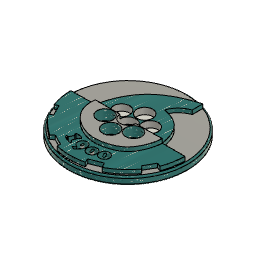
Pin (Autodesk Fusion 360 design; units mm, degrees)
Autodesk Fusion 360 part; units mm, degrees
cylinder "CylinderPrimitive1" add diameter 15 height 1 placed x (1, 0, 0) y (0, 1, 0) z (0, 0, 1) at (0, 0, 0)
fillet "Fillet1" radius 0.2 1 edges at (-6.9925, -2.7121, 1)
fillet "Fillet2" radius 0.2 1 edges at (-6.9925, 2.7121, 0)
shell "Shell1" thickness 0.3 removed faces 0 bodies 1
cylinder "CylinderPrimitive2" cut diameter 2 height 1 placed x (1, 0, 0) y (0, 1, 0) z (0, 0, 1) at (0, 0, 0.3)
cylinder "CylinderPrimitive3" cut diameter 2 height -0.3 placed x (1, 0, 0) y (0, 1, 0) z (0, 0, 1) at (-0.0026, -2.1739, 1)
cylinder "CylinderPrimitive4" cut diameter 2 height -0.3 placed x (1, 0, 0) y (0, 1, 0) z (0, 0, 1) at (-1.832, 1.0276, 1)
cylinder "CylinderPrimitive5" cut diameter 2 height -0.3 placed x (1, 0, 0) y (0, 1, 0) z (0, 0, 1) at (-1.832, -1.0481, 1)
cylinder "CylinderPrimitive6" cut diameter 2 height -0.3 placed x (1, 0, 0) y (0, 1, 0) z (0, 0, 1) at (0, 2.1, 1)
cylinder "CylinderPrimitive7" cut diameter 2 height -0.3 placed x (1, 0, 0) y (0, 1, 0) z (0, 0, 1) at (1.8, 1, 1)
cylinder "CylinderPrimitive8" cut diameter 2 height -0.3 placed x (1, 0, 0) y (0, 1, 0) z (0, 0, 1) at (1.8, -1.1, 1)
cylinder "CylinderPrimitive9" cut diameter 1.25 height -0.3 placed x (1, 0, 0) y (0, 1, 0) z (0, 0, 1) at (1.9983, -4.9501, 1)
sketch "Sketch22" plane through (0, 0, 0.3) normal (0, 0, 1) x (-1, 0, 0)
  circle A0 centre (0, 0) radius 7.2
  ellipse E0 centre (-2.0085, 4.9449) end of major axis (-2.1682, 5.2369) minor radius 0.1458
  line L0 (-1.8488, 4.6529) -> (-2.1682, 5.2369)
  line L1 (-1.8806, 5.0149) -> (-2.1365, 4.8749)
  constraint coincident E0 L0.start
  constraint coincident E0 L0.end
  constraint coincident E0 L1.start
  constraint coincident E0 L1.end
extrude "Extrude1" add sketch "Sketch22" along normal blind 0.7 contours E0 L0 L1 | E0 L0 L1 | E0 L0 L1 | E0 L0 L1
cylinder "CylinderPrimitive10" cut diameter 1.25 height -0.3 placed x (1, 0, 0) y (0, 1, 0) z (0, 0, 1) at (0.7297, -5.2531, 1)
sketch "Sketch24" plane through (0, 0, 0.3) normal (0, 0, 1) x (-1, 0, 0)
  ellipse E0 centre (-2.0085, 4.9449) end of major axis (-2.1682, 5.2369) minor radius 0.1458
  circle A0 centre (0, 0) radius 7.2
  ellipse E1 centre (-0.7296, 5.2552) end of major axis (-0.8009, 5.5528) minor radius 0.1336
  line L0 (-0.6584, 4.9577) -> (-0.8009, 5.5528)
  line L1 (-0.5997, 5.2863) -> (-0.8596, 5.2241)
  constraint coincident E1 L0.start
  constraint coincident E1 L0.end
  constraint coincident E1 L1.start
  constraint coincident E1 L1.end
extrude "Extrude2" add sketch "Sketch24" along normal blind 0.7 contours E1 L0 L1 | E1 L0 L1 | E1 L0 L1 | E1 L0 L1
cylinder "CylinderPrimitive11" cut diameter 1.175 height -0.3 placed x (1, 0, 0) y (0, 1, 0) z (0, 0, 1) at (-0.5634, -5.1632, 1)
sketch "Sketch26" plane through (0, 0, 0.3) normal (0, 0, 1) x (-1, 0, 0)
  ellipse E0 centre (-0.7296, 5.2552) end of major axis (-0.8009, 5.5528) minor radius 0.1336
  ellipse E1 centre (-2.0085, 4.9449) end of major axis (-2.1682, 5.2369) minor radius 0.1458
  circle A0 centre (0, 0) radius 7.2
  ellipse E2 centre (0.5487, 5.1901) end of major axis (0.5487, 5.4) minor radius 0.1259
  line L0 (0.5487, 4.9802) -> (0.5487, 5.4)
  line L1 (0.6746, 5.1901) -> (0.4229, 5.1901)
  constraint vertical L0
  constraint coincident E2 L0.start
  constraint coincident E2 L0.end
  constraint coincident E2 L1.start
  constraint coincident E2 L1.end
extrude "Extrude3" add sketch "Sketch26" along normal blind 0.7 contours E2 L0 L1 | E2 L0 L1 | E2 L0 L1 | E2 L0 L1
sketch "Sketch27" plane through (0, 0, 1) normal (0, 0, 1) x (-1, 0, 0)
  circle A0 centre (0.5634, 5.1632) radius 0.5875
  circle A1 centre (-0.7297, 5.2531) radius 0.625
  circle A2 centre (-1.9983, 4.9501) radius 0.625
  circle A3 centre (-1.8, 1.1) radius 1
  circle A4 centre (-1.8, -1) radius 1
  circle A5 centre (0, -2.1) radius 1
  circle A6 centre (1.832, 1.0481) radius 1
  circle A7 centre (1.832, -1.0276) radius 1
  circle A8 centre (0.0026, 2.1739) radius 1
  circle A9 centre (0, 0) radius 1
  circle A10 centre (0, 0) radius 7.3
  spline S0 degree 5 poles (0.014, 5.3712) (0.023, 5.3959) (0.0414, 5.4447) (0.0703, 5.5157) (0.1114, 5.6061) (0.1671, 5.7113) (0.2276, 5.8082) (0.2934, 5.896) (0.3646, 5.9743) (0.4412, 6.0434) (0.5227, 6.1039) (0.5915, 6.146) (0.645, 6.1743) (0.6815, 6.1917) (0.7, 6.2) knots 0 0 0 0 0 0 0.1 0.2 0.3 0.4 0.5 0.6 0.7 0.8 0.9 1 1 1 1 1 1
  spline S1 degree 5 poles (0.7, 5.7346) (0.7041, 5.7419) (0.7123, 5.7564) (0.7253, 5.7775) (0.7435, 5.8047) (0.7682, 5.8367) (0.7949, 5.8666) (0.8238, 5.8943) (0.8549, 5.9197) (0.8882, 5.9428) (0.9235, 5.9639) (0.9533, 5.9792) (0.9763, 5.9899) (0.9921, 5.9967) (1, 6) knots 0 0 0 0 0 0 0.1 0.2 0.3 0.4 0.5 0.6 0.7 0.8 0.9 1 1 1 1 1 1
  line L0 (0.7, 6.2) -> (1, 6)
  point P0 (0.3, 5.9)
  point P1 (0.8243, 5.8937)
  constraint coincident A0 S0.start
  constraint coincident A0 S1.start
extrude "Extrude4" cut sketch "Sketch27" against normal blind 0.3 contours A0 S0 S1 L0
sketch "Sketch28" plane through (0, 0, 1) normal (0, 0, 1) x (-1, 0, 0)
  spline S0 degree 5 poles (1, 6) (0.9921, 5.9967) (0.9763, 5.9899) (0.9533, 5.9792) (0.9235, 5.9639) (0.8882, 5.9428) (0.8549, 5.9197) (0.8238, 5.8943) (0.7949, 5.8666) (0.7682, 5.8367) (0.7435, 5.8047) (0.7253, 5.7775) (0.7123, 5.7564) (0.7041, 5.7419) (0.7, 5.7346) knots -1 -1 -1 -1 -1 -1 -0.9 -0.8 -0.7 -0.6 -0.5 -0.4 -0.3 -0.2 -0.1 0 0 0 0 0 0
  arc A0 (0.014, 5.3712) -> (0.7, 5.7346) centre (0.5634, 5.1632) ccw
  spline S1 degree 5 poles (0.014, 5.3712) (0.023, 5.3959) (0.0414, 5.4447) (0.0703, 5.5157) (0.1114, 5.6061) (0.1671, 5.7113) (0.2276, 5.8082) (0.2934, 5.896) (0.3646, 5.9743) (0.4412, 6.0434) (0.5227, 6.1039) (0.5915, 6.146) (0.645, 6.1743) (0.6815, 6.1917) (0.7, 6.2) knots 0 0 0 0 0 0 0.1 0.2 0.3 0.4 0.5 0.6 0.7 0.8 0.9 1 1 1 1 1 1
  line L0 (0.7, 6.2) -> (1, 6)
  circle A1 centre (-0.7297, 5.2531) radius 0.625
  circle A2 centre (-1.9983, 4.9501) radius 0.625
  circle A3 centre (-1.8, 1.1) radius 1
  circle A4 centre (-1.8, -1) radius 1
  circle A5 centre (0, -2.1) radius 1
  circle A6 centre (1.832, 1.0481) radius 1
  circle A7 centre (1.832, -1.0276) radius 1
  circle A8 centre (0.0026, 2.1739) radius 1
  circle A9 centre (0, 0) radius 1
  circle A10 centre (0, 0) radius 7.3
  spline S2 degree 5 poles (2.1731, 4.3495) (2.1626, 4.3461) (2.1405, 4.3398) (2.1042, 4.3322) (2.0494, 4.3261) (1.9705, 4.325) (1.8818, 4.3305) (1.785, 4.3423) (1.6831, 4.3601) (1.5808, 4.3831) (1.4843, 4.4103) (1.3999, 4.4405) (1.3336, 4.4724) (1.2892, 4.5048) (1.2683, 4.5365) (1.2686, 4.5667) (1.2857, 4.5947) (1.3144, 4.6201) (1.3495, 4.6426) (1.3872, 4.6619) (1.4255, 4.6781) (1.4557, 4.6884) (1.478, 4.6948) (1.4927, 4.6984) (1.5, 4.7) knots 0 0 0 0 0 0 0.05 0.1 0.15 0.2 0.25 0.3 0.35 0.4 0.45 0.5 0.55 0.6 0.65 0.7 0.75 0.8 0.85 0.9 0.95 1 1 1 1 1 1
  line L1 (1.5, 4.7) -> (1.7, 5.3)
  spline S3 degree 5 poles (1.7, 5.3) (1.7086, 5.3088) (1.7237, 5.3259) (1.7404, 5.3504) (1.7508, 5.3807) (1.7442, 5.4149) (1.7194, 5.4456) (1.6794, 5.4737) (1.6295, 5.5008) (1.5772, 5.5288) (1.5309, 5.5592) (1.4986, 5.5926) (1.4873, 5.628) (1.5016, 5.6619) (1.5434, 5.6892) (1.6127, 5.7046) (1.7069, 5.7036) (1.8216, 5.6836) (1.95, 5.6454) (2.084, 5.592) (2.2151, 5.5276) (2.3346, 5.4577) (2.4346, 5.3876) (2.5084, 5.3218) (2.5517, 5.2637) (2.5622, 5.2152) (2.5436, 5.1847) (2.5144, 5.1665) (2.4882, 5.1565) (2.4734, 5.1521) knots 0 0 0 0 0 0 0.04 0.08 0.12 0.16 0.2 0.24 0.28 0.32 0.36 0.4 0.44 0.48 0.52 0.56 0.6 0.64 0.68 0.72 0.76 0.8 0.84 0.88 0.92 0.96 1 1 1 1 1 1
  line L2 (2.4734, 5.1521) -> (2.3, 5.2)
  line L3 (2.3, 5.2) -> (2.0366, 4.6553)
  spline S4 degree 5 poles (2.0366, 4.6553) (2.0437, 4.6504) (2.0575, 4.6406) (2.0771, 4.6256) (2.1009, 4.6049) (2.1265, 4.5778) (2.1476, 4.5493) (2.1638, 4.5195) (2.1749, 4.4882) (2.1811, 4.4555) (2.1828, 4.4214) (2.1809, 4.3932) (2.1777, 4.3716) (2.1748, 4.3569) (2.1731, 4.3495) knots 0 0 0 0 0 0 0.1 0.2 0.3 0.4 0.5 0.6 0.7 0.8 0.9 1 1 1 1 1 1
  point P0 (1.7473, 4.3495)
  point P1 (1.3, 4.5)
  point P2 (1.3269, 4.6272)
  point P3 (1.7, 5.4578)
  point P4 (1.5, 5.6)
  point P5 (1.7, 5.7)
  point P6 (2.457, 5.365)
  point P7 (2.1627, 4.5186)
extrude "Extrude5" cut sketch "Sketch28" against normal blind 0.3 contours S2 L1 S3 L2 L3 S4
sketch "Sketch29" plane through (0, 0, 1) normal (0, 0, 1) x (-1, 0, 0)
  line L0 (2.4734, 5.1521) -> (2.3, 5.2)
  line L1 (2.3, 5.2) -> (2.0366, 4.6553)
  spline S0 degree 5 poles (2.0366, 4.6553) (2.0437, 4.6504) (2.0575, 4.6406) (2.0771, 4.6256) (2.1009, 4.6049) (2.1265, 4.5778) (2.1476, 4.5493) (2.1638, 4.5195) (2.1749, 4.4882) (2.1811, 4.4555) (2.1828, 4.4214) (2.1809, 4.3932) (2.1777, 4.3716) (2.1748, 4.3569) (2.1731, 4.3495) knots 0 0 0 0 0 0 0.1 0.2 0.3 0.4 0.5 0.6 0.7 0.8 0.9 1 1 1 1 1 1
  spline S1 degree 5 poles (2.1731, 4.3495) (2.1626, 4.3461) (2.1405, 4.3398) (2.1042, 4.3322) (2.0494, 4.3261) (1.9705, 4.325) (1.8818, 4.3305) (1.785, 4.3423) (1.6831, 4.3601) (1.5808, 4.3831) (1.4843, 4.4103) (1.3999, 4.4405) (1.3336, 4.4724) (1.2892, 4.5048) (1.2683, 4.5365) (1.2686, 4.5667) (1.2857, 4.5947) (1.3144, 4.6201) (1.3495, 4.6426) (1.3872, 4.6619) (1.4255, 4.6781) (1.4557, 4.6884) (1.478, 4.6948) (1.4927, 4.6984) (1.5, 4.7) knots 0 0 0 0 0 0 0.05 0.1 0.15 0.2 0.25 0.3 0.35 0.4 0.45 0.5 0.55 0.6 0.65 0.7 0.75 0.8 0.85 0.9 0.95 1 1 1 1 1 1
  line L2 (1.5, 4.7) -> (1.7, 5.3)
  spline S2 degree 5 poles (1.7, 5.3) (1.7086, 5.3088) (1.7237, 5.3259) (1.7404, 5.3504) (1.7508, 5.3807) (1.7442, 5.4149) (1.7194, 5.4456) (1.6794, 5.4737) (1.6295, 5.5008) (1.5772, 5.5288) (1.5309, 5.5592) (1.4986, 5.5926) (1.4873, 5.628) (1.5016, 5.6619) (1.5434, 5.6892) (1.6127, 5.7046) (1.7069, 5.7036) (1.8216, 5.6836) (1.95, 5.6454) (2.084, 5.592) (2.2151, 5.5276) (2.3346, 5.4577) (2.4346, 5.3876) (2.5084, 5.3218) (2.5517, 5.2637) (2.5622, 5.2152) (2.5436, 5.1847) (2.5144, 5.1665) (2.4882, 5.1565) (2.4734, 5.1521) knots 0 0 0 0 0 0 0.04 0.08 0.12 0.16 0.2 0.24 0.28 0.32 0.36 0.4 0.44 0.48 0.52 0.56 0.6 0.64 0.68 0.72 0.76 0.8 0.84 0.88 0.92 0.96 1 1 1 1 1 1
  spline S3 degree 5 poles (1, 6) (0.9921, 5.9967) (0.9763, 5.9899) (0.9533, 5.9792) (0.9235, 5.9639) (0.8882, 5.9428) (0.8549, 5.9197) (0.8238, 5.8943) (0.7949, 5.8666) (0.7682, 5.8367) (0.7435, 5.8047) (0.7253, 5.7775) (0.7123, 5.7564) (0.7041, 5.7419) (0.7, 5.7346) knots -1 -1 -1 -1 -1 -1 -0.9 -0.8 -0.7 -0.6 -0.5 -0.4 -0.3 -0.2 -0.1 0 0 0 0 0 0
  arc A0 (0.014, 5.3712) -> (0.7, 5.7346) centre (0.5634, 5.1632) ccw
  spline S4 degree 5 poles (0.014, 5.3712) (0.023, 5.3959) (0.0414, 5.4447) (0.0703, 5.5157) (0.1114, 5.6061) (0.1671, 5.7113) (0.2276, 5.8082) (0.2934, 5.896) (0.3646, 5.9743) (0.4412, 6.0434) (0.5227, 6.1039) (0.5915, 6.146) (0.645, 6.1743) (0.6815, 6.1917) (0.7, 6.2) knots 0 0 0 0 0 0 0.1 0.2 0.3 0.4 0.5 0.6 0.7 0.8 0.9 1 1 1 1 1 1
  line L3 (0.7, 6.2) -> (1, 6)
  circle A1 centre (-0.7297, 5.2531) radius 0.625
  circle A2 centre (-1.9983, 4.9501) radius 0.625
  circle A3 centre (-1.8, 1.1) radius 1
  circle A4 centre (-1.8, -1) radius 1
  circle A5 centre (0, -2.1) radius 1
  circle A6 centre (1.832, 1.0481) radius 1
  circle A7 centre (1.832, -1.0276) radius 1
  circle A8 centre (0.0026, 2.1739) radius 1
  circle A9 centre (0, 0) radius 1
  circle A10 centre (0, 0) radius 7.3
  spline S5 degree 5 poles (4.13, -0.0103) (4.0869, -0.2194) (3.9925, -0.6311) (3.8269, -1.2295) (3.5572, -1.9883) (3.1331, -2.8673) (2.6146, -3.6709) (1.9943, -4.3931) (1.2689, -5.0314) (0.4435, -5.5897) (-0.4741, -6.0744) (-1.2757, -6.4081) (-1.9125, -6.63) (-2.3525, -6.7656) (-2.5765, -6.8302) knots 0 0 0 0 0 0 0.1 0.2 0.3 0.4 0.5 0.6 0.7 0.8 0.9 1 1 1 1 1 1
  line L4 (-2.5765, -6.8302) -> (-2.5765, -5.5)
  spline S6 degree 5 poles (-2.5765, -5.5) (-2.5232, -5.4786) (-2.4184, -5.4346) (-2.266, -5.3651) (-2.0727, -5.2656) (-1.8485, -5.1288) (-1.6435, -4.9784) (-1.4591, -4.8134) (-1.2965, -4.633) (-1.1549, -4.4377) (-1.0327, -4.2287) (-0.9493, -4.0513) (-0.8943, -3.913) (-0.8609, -3.8184) (-0.845, -3.7705) knots 0 0 0 0 0 0 0.1 0.2 0.3 0.4 0.5 0.6 0.7 0.8 0.9 1 1 1 1 1 1
  spline S7 degree 5 poles (-0.845, -3.7705) (-0.9645, -3.747) (-1.1989, -3.6953) (-1.5374, -3.6041) (-1.9618, -3.4547) (-2.4443, -3.2186) (-2.8747, -2.9286) (-3.2489, -2.5806) (-3.5648, -2.1724) (-3.8249, -1.7066) (-4.0335, -1.1877) (-4.1627, -0.7337) (-4.2397, -0.3726) (-4.2824, -0.1229) (-4.3015, 0.0041) knots 0 0 0 0 0 0 0.1 0.2 0.3 0.4 0.5 0.6 0.7 0.8 0.9 1 1 1 1 1 1
  line L5 (-4.3015, 0.0041) -> (-7.1651, 0.0041)
  spline S8 degree 5 poles (-7.1651, 0.0041) (-7.1621, 0.0669) (-7.1557, 0.1917) (-7.1441, 0.3763) (-7.125, 0.6172) (-7.0942, 0.9092) (-7.0561, 1.191) (-7.01, 1.4618) (-6.9555, 1.7211) (-6.8927, 1.969) (-6.8222, 2.2065) (-6.7602, 2.3887) (-6.7107, 2.5213) (-6.6764, 2.6079) (-6.6589, 2.6507) knots 0 0 0 0 0 0 0.1 0.2 0.3 0.4 0.5 0.6 0.7 0.8 0.9 1 1 1 1 1 1
  line L6 (-6.6589, 2.6507) -> (-6.1816, 2.4772)
  line L7 (-6.1816, 2.4772) -> (-5.473, 3.7354)
  line L8 (-5.473, 3.7354) -> (-5.8273, 4.1259)
  spline S9 degree 5 poles (-5.8273, 4.1259) (-5.7769, 4.187) (-5.6759, 4.3077) (-5.5236, 4.4848) (-5.3192, 4.7127) (-5.0612, 4.9829) (-4.8005, 5.2371) (-4.5368, 5.4739) (-4.2699, 5.6923) (-4, 5.8929) (-3.7272, 6.0769) (-3.5069, 6.2118) (-3.3406, 6.3066) (-3.2293, 6.367) (-3.1735, 6.3965) knots 0 0 0 0 0 0 0.1 0.2 0.3 0.4 0.5 0.6 0.7 0.8 0.9 1 1 1 1 1 1
  line L9 (-3.1735, 6.3965) -> (-2.8264, 5.8035)
  line L10 (-2.8264, 5.8035) -> (-1.3367, 6.3965)
  line L11 (-1.3367, 6.3965) -> (-1.5394, 6.9057)
  spline S10 degree 5 poles (-1.5394, 6.9057) (-1.4688, 6.9219) (-1.3277, 6.9529) (-1.1159, 6.9952) (-0.8336, 7.043) (-0.4807, 7.0873) (-0.1277, 7.1149) (0.2252, 7.1243) (0.5781, 7.1149) (0.931, 7.0873) (1.2838, 7.043) (1.5662, 6.9952) (1.7779, 6.9529) (1.919, 6.9219) (1.9896, 6.9057) knots 0 0 0 0 0 0 0.1 0.2 0.3 0.4 0.5 0.6 0.7 0.8 0.9 1 1 1 1 1 1
  line L12 (1.9896, 6.9057) -> (1.9896, 6.5)
  line L13 (1.9896, 6.5) -> (3.2912, 5.8469)
  line L14 (3.2912, 5.8469) -> (3.6817, 6.1735)
  spline S11 degree 5 poles (3.6817, 6.1735) (3.7466, 6.1256) (3.8748, 6.0303) (4.0624, 5.8884) (4.3029, 5.7015) (4.5865, 5.472) (4.8512, 5.2469) (5.0953, 5.0266) (5.3175, 4.8115) (5.5182, 4.6016) (5.6985, 4.3964) (5.8279, 4.2358) (5.917, 4.1172) (5.9729, 4.0389) (6, 4) knots 0 0 0 0 0 0 0.1 0.2 0.3 0.4 0.5 0.6 0.7 0.8 0.9 1 1 1 1 1 1
  line L15 (6, 4) -> (5.5907, 3.7354)
  line L16 (5.5907, 3.7354) -> (6.2849, 2.3904)
  line L17 (6.2849, 2.3904) -> (6.6861, 2.5975)
  spline S12 degree 5 poles (6.6861, 2.5975) (6.705, 2.5422) (6.7421, 2.432) (6.7951, 2.2677) (6.8608, 2.0505) (6.9339, 1.7825) (6.9971, 1.5182) (7.0496, 1.2581) (7.0909, 1.0023) (7.1213, 0.7506) (7.1415, 0.5029) (7.1503, 0.3075) (7.153, 0.1625) (7.1531, 0.0664) (7.1527, 0.0186) knots 0 0 0 0 0 0 0.1 0.2 0.3 0.4 0.5 0.6 0.7 0.8 0.9 1 1 1 1 1 1
  line L18 (7.1527, 0.0186) -> (4.13, -0.0103)
  point P0 (2.033, -4.3057)
  point P1 (-1.4524, -4.7974)
  point P2 (-3.2168, -2.5846)
  point P3 (-7, 1.5)
  point P4 (-4.5, 5.5)
  point P5 (0.2252, 7.1196)
  point P6 (5.1569, 4.9647)
  point P7 (7.0514, 1.2334)
  constraint coincident A10 S5.end
  constraint vertical L4
  constraint horizontal L5
  constraint perpendicular L10 L11
  constraint vertical L12
  constraint perpendicular L16 L17
extrude "Extrude6" add sketch "Sketch29" along normal blind 0.5 contours S5 L4 S6 S7 L5 S8 L6 L7 L8 S9 L9 L10 L11 S10 L12 L13 L14 S11 L15 L16 L17 S12 L18
extrude "Extrude7" add 1 faces at (-0.5898, -5.2144, 1) along direction (0, 0, 1) blind 0.5
extrude "Extrude8" add 1 faces at (0.697, -5.3058, 1) along direction (0, 0, 1) blind 0.5
extrude "Extrude9" add 1 faces at (2.0285, -4.8824, 1) along direction (0, 0, 1) blind 0.5
sketch "Sketch31" plane through (0, 0, 1.5) normal (0, 0, 1) x (-1, 0, 0)
  arc A0 (0.014, 5.3712) -> (0.7, 5.7346) centre (0.5634, 5.1632) ccw
  spline S0 degree 5 poles (0.014, 5.3712) (0.023, 5.3959) (0.0414, 5.4447) (0.0703, 5.5157) (0.1114, 5.6061) (0.1671, 5.7113) (0.2276, 5.8082) (0.2934, 5.896) (0.3646, 5.9743) (0.4412, 6.0434) (0.5227, 6.1039) (0.5915, 6.146) (0.645, 6.1743) (0.6815, 6.1917) (0.7, 6.2) knots 0 0 0 0 0 0 0.1 0.2 0.3 0.4 0.5 0.6 0.7 0.8 0.9 1 1 1 1 1 1
  line L0 (0.7, 6.2) -> (1, 6)
  spline S1 degree 5 poles (1, 6) (0.9921, 5.9967) (0.9763, 5.9899) (0.9533, 5.9792) (0.9235, 5.9639) (0.8882, 5.9428) (0.8549, 5.9197) (0.8238, 5.8943) (0.7949, 5.8666) (0.7682, 5.8367) (0.7435, 5.8047) (0.7253, 5.7775) (0.7123, 5.7564) (0.7041, 5.7419) (0.7, 5.7346) knots -1 -1 -1 -1 -1 -1 -0.9 -0.8 -0.7 -0.6 -0.5 -0.4 -0.3 -0.2 -0.1 0 0 0 0 0 0
  circle A1 centre (0, 0) radius 1
  line L1 (1.5, 4.7) -> (1.7, 5.3)
  spline S2 degree 5 poles (1.7, 5.3) (1.7086, 5.3088) (1.7237, 5.3259) (1.7404, 5.3504) (1.7508, 5.3807) (1.7442, 5.4149) (1.7194, 5.4456) (1.6794, 5.4737) (1.6295, 5.5008) (1.5772, 5.5288) (1.5309, 5.5592) (1.4986, 5.5926) (1.4873, 5.628) (1.5016, 5.6619) (1.5434, 5.6892) (1.6127, 5.7046) (1.7069, 5.7036) (1.8216, 5.6836) (1.95, 5.6454) (2.084, 5.592) (2.2151, 5.5276) (2.3346, 5.4577) (2.4346, 5.3876) (2.5084, 5.3218) (2.5517, 5.2637) (2.5622, 5.2152) (2.5436, 5.1847) (2.5144, 5.1665) (2.4882, 5.1565) (2.4734, 5.1521) knots 0 0 0 0 0 0 0.04 0.08 0.12 0.16 0.2 0.24 0.28 0.32 0.36 0.4 0.44 0.48 0.52 0.56 0.6 0.64 0.68 0.72 0.76 0.8 0.84 0.88 0.92 0.96 1 1 1 1 1 1
  line L2 (2.4734, 5.1521) -> (2.3, 5.2)
  line L3 (2.3, 5.2) -> (2.0366, 4.6553)
  spline S3 degree 5 poles (2.0366, 4.6553) (2.0437, 4.6504) (2.0575, 4.6406) (2.0771, 4.6256) (2.1009, 4.6049) (2.1265, 4.5778) (2.1476, 4.5493) (2.1638, 4.5195) (2.1749, 4.4882) (2.1811, 4.4555) (2.1828, 4.4214) (2.1809, 4.3932) (2.1777, 4.3716) (2.1748, 4.3569) (2.1731, 4.3495) knots 0 0 0 0 0 0 0.1 0.2 0.3 0.4 0.5 0.6 0.7 0.8 0.9 1 1 1 1 1 1
  spline S4 degree 5 poles (2.1731, 4.3495) (2.1626, 4.3461) (2.1405, 4.3398) (2.1042, 4.3322) (2.0494, 4.3261) (1.9705, 4.325) (1.8818, 4.3305) (1.785, 4.3423) (1.6831, 4.3601) (1.5808, 4.3831) (1.4843, 4.4103) (1.3999, 4.4405) (1.3336, 4.4724) (1.2892, 4.5048) (1.2683, 4.5365) (1.2686, 4.5667) (1.2857, 4.5947) (1.3144, 4.6201) (1.3495, 4.6426) (1.3872, 4.6619) (1.4255, 4.6781) (1.4557, 4.6884) (1.478, 4.6948) (1.4927, 4.6984) (1.5, 4.7) knots 0 0 0 0 0 0 0.05 0.1 0.15 0.2 0.25 0.3 0.35 0.4 0.45 0.5 0.55 0.6 0.65 0.7 0.75 0.8 0.85 0.9 0.95 1 1 1 1 1 1
  circle A2 centre (1.832, -1.0276) radius 1
  circle A3 centre (-1.9983, 4.9501) radius 0.625
  circle A4 centre (0, -2.1) radius 1
  circle A5 centre (0.0026, 2.1739) radius 1
  circle A6 centre (-1.8, 1.1) radius 1
  circle A7 centre (1.832, 1.0481) radius 1
  circle A8 centre (-1.8, -1) radius 1
  circle A9 centre (-0.7297, 5.2531) radius 0.625
  spline S5 degree 5 poles (7.1527, 0.0186) (7.1531, 0.0664) (7.153, 0.1625) (7.1503, 0.3075) (7.1415, 0.5029) (7.1213, 0.7506) (7.0909, 1.0023) (7.0496, 1.2581) (6.9971, 1.5182) (6.9339, 1.7825) (6.8608, 2.0505) (6.7951, 2.2677) (6.7421, 2.432) (6.705, 2.5422) (6.6861, 2.5975) knots -1 -1 -1 -1 -1 -1 -0.9 -0.8 -0.7 -0.6 -0.5 -0.4 -0.3 -0.2 -0.1 0 0 0 0 0 0
  line L4 (6.6861, 2.5975) -> (6.2849, 2.3904)
  line L5 (6.2849, 2.3904) -> (5.5907, 3.7354)
  line L6 (5.5907, 3.7354) -> (6, 4)
  spline S6 degree 5 poles (6, 4) (5.9729, 4.0389) (5.917, 4.1172) (5.8279, 4.2358) (5.6985, 4.3964) (5.5182, 4.6016) (5.3175, 4.8115) (5.0953, 5.0266) (4.8512, 5.2469) (4.5865, 5.472) (4.3029, 5.7015) (4.0624, 5.8884) (3.8748, 6.0303) (3.7466, 6.1256) (3.6817, 6.1735) knots -1 -1 -1 -1 -1 -1 -0.9 -0.8 -0.7 -0.6 -0.5 -0.4 -0.3 -0.2 -0.1 0 0 0 0 0 0
  line L7 (3.6817, 6.1735) -> (3.2912, 5.8469)
  line L8 (3.2912, 5.8469) -> (1.9896, 6.5)
  line L9 (1.9896, 6.5) -> (1.9896, 6.9057)
  spline S7 degree 5 poles (1.9896, 6.9057) (1.919, 6.9219) (1.7779, 6.9529) (1.5662, 6.9952) (1.2838, 7.043) (0.931, 7.0873) (0.5781, 7.1149) (0.2252, 7.1243) (-0.1277, 7.1149) (-0.4807, 7.0873) (-0.8336, 7.043) (-1.1159, 6.9952) (-1.3277, 6.9529) (-1.4688, 6.9219) (-1.5394, 6.9057) knots -1 -1 -1 -1 -1 -1 -0.9 -0.8 -0.7 -0.6 -0.5 -0.4 -0.3 -0.2 -0.1 0 0 0 0 0 0
  line L10 (-1.5394, 6.9057) -> (-1.3367, 6.3965)
  line L11 (-1.3367, 6.3965) -> (-2.8264, 5.8035)
  line L12 (-2.8264, 5.8035) -> (-3.1735, 6.3965)
  spline S8 degree 5 poles (-3.1735, 6.3965) (-3.2293, 6.367) (-3.3406, 6.3066) (-3.5069, 6.2118) (-3.7272, 6.0769) (-4, 5.8929) (-4.2699, 5.6923) (-4.5368, 5.4739) (-4.8005, 5.2371) (-5.0612, 4.9829) (-5.3192, 4.7127) (-5.5236, 4.4848) (-5.6759, 4.3077) (-5.7769, 4.187) (-5.8273, 4.1259) knots -1 -1 -1 -1 -1 -1 -0.9 -0.8 -0.7 -0.6 -0.5 -0.4 -0.3 -0.2 -0.1 0 0 0 0 0 0
  line L13 (-5.8273, 4.1259) -> (-5.473, 3.7354)
  line L14 (-5.473, 3.7354) -> (-6.1816, 2.4772)
  line L15 (-6.1816, 2.4772) -> (-6.6589, 2.6507)
  spline S9 degree 5 poles (-6.6589, 2.6507) (-6.6764, 2.6079) (-6.7107, 2.5213) (-6.7602, 2.3887) (-6.8222, 2.2065) (-6.8927, 1.969) (-6.9555, 1.7211) (-7.01, 1.4618) (-7.0561, 1.191) (-7.0942, 0.9092) (-7.125, 0.6172) (-7.1441, 0.3763) (-7.1557, 0.1917) (-7.1621, 0.0669) (-7.1651, 0.0041) knots -1 -1 -1 -1 -1 -1 -0.9 -0.8 -0.7 -0.6 -0.5 -0.4 -0.3 -0.2 -0.1 0 0 0 0 0 0
  line L16 (-7.1651, 0.0041) -> (-4.3015, 0.0041)
  spline S10 degree 5 poles (-4.3015, 0.0041) (-4.2824, -0.1229) (-4.2397, -0.3726) (-4.1627, -0.7337) (-4.0335, -1.1877) (-3.8249, -1.7066) (-3.5648, -2.1724) (-3.2489, -2.5806) (-2.8747, -2.9286) (-2.4443, -3.2186) (-1.9618, -3.4547) (-1.5374, -3.6041) (-1.1989, -3.6953) (-0.9645, -3.747) (-0.845, -3.7705) knots -1 -1 -1 -1 -1 -1 -0.9 -0.8 -0.7 -0.6 -0.5 -0.4 -0.3 -0.2 -0.1 0 0 0 0 0 0
  spline S11 degree 5 poles (-0.845, -3.7705) (-0.8609, -3.8184) (-0.8943, -3.913) (-0.9493, -4.0513) (-1.0327, -4.2287) (-1.1549, -4.4377) (-1.2965, -4.633) (-1.4591, -4.8134) (-1.6435, -4.9784) (-1.8485, -5.1288) (-2.0727, -5.2656) (-2.266, -5.3651) (-2.4184, -5.4346) (-2.5232, -5.4786) (-2.5765, -5.5) knots -1 -1 -1 -1 -1 -1 -0.9 -0.8 -0.7 -0.6 -0.5 -0.4 -0.3 -0.2 -0.1 0 0 0 0 0 0
  line L17 (-2.5765, -5.5) -> (-2.5765, -6.8302)
  spline S12 degree 5 poles (-2.5765, -6.8302) (-2.3525, -6.7656) (-1.9125, -6.63) (-1.2757, -6.4081) (-0.4741, -6.0744) (0.4435, -5.5897) (1.2689, -5.0314) (1.9943, -4.3931) (2.6146, -3.6709) (3.1331, -2.8673) (3.5572, -1.9883) (3.8269, -1.2295) (3.9925, -0.6311) (4.0869, -0.2194) (4.13, -0.0103) knots -1 -1 -1 -1 -1 -1 -0.9 -0.8 -0.7 -0.6 -0.5 -0.4 -0.3 -0.2 -0.1 0 0 0 0 0 0
  line L18 (4.13, -0.0103) -> (7.1527, 0.0186)
  spline S13 degree 5 poles (4.13, -0.0103) (4.138, 0.0579) (4.1511, 0.1939) (4.1619, 0.3965) (4.1587, 0.6641) (4.1249, 0.994) (4.06, 1.3193) (3.9618, 1.64) (3.8268, 1.9559) (3.6502, 2.2666) (3.4278, 2.5711) (3.1571, 2.8671) (2.8385, 3.1508) (2.477, 3.4159) (2.0822, 3.6545) (1.6658, 3.8583) (1.2399, 4.0197) (0.8157, 4.1335) (0.4013, 4.1978) (-0.0001, 4.2157) (-0.389, 4.1934) (-0.7679, 4.1388) (-1.1396, 4.0585) (-1.5059, 3.9568) (-1.8652, 3.8328) (-2.2134, 3.6814) (-2.545, 3.4964) (-2.8542, 3.2722) (-3.1358, 3.0063) (-3.3868, 2.7019) (-3.6059, 2.3672) (-3.7933, 2.0129) (-3.95, 1.6508) (-4.0772, 1.2918) (-4.1761, 0.9438) (-4.2473, 0.6112) (-4.2824, 0.3592) (-4.2967, 0.1785) (-4.3008, 0.0616) (-4.3015, 0.0041) knots 0 0 0 0 0 0 0.028571 0.057143 0.085714 0.114286 0.142857 0.171429 0.2 0.228571 0.257143 0.285714 0.314286 0.342857 0.371429 0.4 0.428571 0.457143 0.485714 0.514286 0.542857 0.571429 0.6 0.628571 0.657143 0.685714 0.714286 0.742857 0.771429 0.8 0.828571 0.857143 0.885714 0.914286 0.942857 0.971429 1 1 1 1 1 1
  line L19 (4.13, -0.0103) -> (0, 0)
  spline S14 degree 5 poles (-4.3015, 0.0041) (-4.1983, 0.0058) (-3.9932, 0.0089) (-3.69, 0.0133) (-3.2947, 0.0181) (-2.8166, 0.0225) (-2.3559, 0.0252) (-1.9145, 0.0259) (-1.4933, 0.0246) (-1.0922, 0.0212) (-0.7099, 0.016) (-0.4178, 0.0104) (-0.2061, 0.0055) (-0.0682, 0.0019) (0, 0) knots 0 0 0 0 0 0 0.1 0.2 0.3 0.4 0.5 0.6 0.7 0.8 0.9 1 1 1 1 1 1
  point P0 (4, 1.5)
  point P1 (3, 3)
  point P2 (0.7546, 4.1342)
  point P3 (-1.2439, 4.0261)
  point P4 (-2.9318, 3.1889)
  point P5 (-4, 1.5)
  point P6 (-1.8054, 0.0252)
  constraint coincident S12.end L18.start
  constraint coincident L16.end S10.start
  constraint coincident A1.centre L19.end
extrude "Extrude10" add sketch "Sketch31" along normal blind 0.5 contours A1 L19 S14 | A1 S13 L19 S14 picked at (-0.2809, 0.6026)
extrude "Extrude11" cut 1 faces at (0.2809, -0.6026, 1.5) along direction (0, 0, 1) blind 0.6
